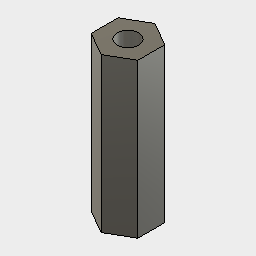
AssemblySpacer18 v2 (Autodesk Fusion 360 archive; units mm, degrees)
design "Spacer M3x18"
Autodesk Fusion 360 part; units mm, degrees
sketch "Sketch1" plane through (0, 0, 0) normal (0, 1, 0) x (1, 0, 0)
  line L0 (2.725, 1.5733) -> (0, 3.1466)
  line L1 (0, 3.1466) -> (-2.725, 1.5733)
  line L2 (-2.725, 1.5733) -> (-2.725, -1.5733)
  line L3 (-2.725, -1.5733) -> (0, -3.1466)
  line L4 (0, -3.1466) -> (2.725, -1.5733)
  line L5 (2.725, -1.5733) -> (2.725, 1.5733)
  circle A0 centre (0, 0) radius 1.25
  dimension "d1" = 2.5
  measures "d1" diameter of A0
extrude "Extrude1" add sketch "Sketch1" along normal blind 18
